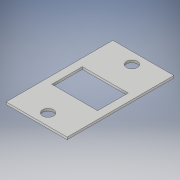
# Autodesk Inventor part: came2
Saved by Autodesk Inventor 2019 (Build 230136000, 136)
## iProperties
Created: 2021-11-18
Part Number: came2
Material: 一般
Document SubType Name: Sheet Metal
Designer: yuta
Density: 1 g/cm^3
Sheet Metal Rule: Default_mm
Appearance: 既定
Author: yuta
Autodesk Inventor part; units mm, degrees
ref_plane "YZ Plane" through (0, 0, 0) normal (1, 0, 0) x (0, 1, 0)
ref_plane "XZ Plane" through (0, 0, 0) normal (0, 1, 0) x (-1, 0, 0)
ref_plane "XY Plane" through (0, 0, 0) normal (0, 0, 1) x (1, 0, 0)
sketch "スケッチ1" plane through (0, 0, 0) normal (0, 1, 0) x (-1, 0, 0)
  line L0 (7.3003, 15.1278) -> (-72.6997, 15.1278)
  line L1 (-72.6997, 15.1278) -> (-72.6997, -124.8722)
  line L2 (-72.6997, -124.8722) -> (7.3003, -124.8722)
  line L3 (7.3003, -124.8722) -> (7.3003, 15.1278)
  point P0 (0, 0)
  dimension "d0" = 80
  dimension "d1" = 140
  constraints: 8 end point, 2 parallel, 1 horizontal, 1 perpendicular
  measures "d0" distance of L2.end L1.end
  measures "d1" distance of L1.end L0.end
extrude "押し出し1" add sketch "スケッチ1" along normal blind 3
sketch "スケッチ2" plane through (0, 3, 0) normal (0, 1, 0) x (1, 0, 0)
  line L0 (2.6997, 34.8722) -> (62.6997, 34.8722)
  line L1 (62.6997, 34.8722) -> (62.6997, 74.8722)
  line L2 (62.6997, 74.8722) -> (2.6997, 74.8722)
  line L3 (2.6997, 74.8722) -> (2.6997, 34.8722)
  circle A0 centre (32.6997, -0.1278) radius 7.15
  circle A1 centre (32.6997, 109.8722) radius 7.15
  line L4 (-7.3003, -15.1278) -> (72.6997, -15.1278) projected
  line L5 (72.6997, 124.8722) -> (-7.3003, 124.8722) projected
  line L6 (-7.3003, 124.8722) -> (-7.3003, -15.1278) projected
  point P0 (0, 0)
  dimension "d4" = 60
  dimension "d5" = 40
  dimension "d6" = 14.3
  dimension "d7" = 14.3
  dimension "d8" = 15
  dimension "d9" = 15
  dimension "d10" = 40
  dimension "d11" = 40
  dimension "d12" = 10
  dimension "d13" = 50
  constraints: 8 end point, 2 centre point, 2 parallel, 1 horizontal, 1 perpendicular
  measures "d4" distance of L2.end L1.end
  measures "d5" distance of L1.end L0.end
  measures "d6" diameter of A0
  measures "d7" diameter of A1
  measures "d8" distance from line of L4 A0.centre
  measures "d9" distance from line of L5 A1.centre
  measures "d10" distance from line of L6 A1.centre
  measures "d11" distance from line of L6 A0.centre
  measures "d12" distance between parallel lines of L6 L3
  measures "d13" distance between parallel lines of L4 L0
extrude "押し出し2" cut sketch "スケッチ2" against normal blind 3
equation "\"BendRadius\" = Thickness"
equation "\"BendReliefWidth\" = Thickness"
equation "\"BendReliefDepth\" = 0.5 * Thickness"
equation "\"CornerReliefSize\" = 4 * Thickness"
equation "\"MinimumRemnant\" = 2 * Thickness"
equation "\"TransitionRadius\" = BendRadius"
equation "\"JacobiRadiusSize\" = BendRadius"
equation "\"GapSize\" = Thickness"
equation "\"Thickness\" = 0.5"
